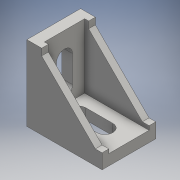
# Autodesk Inventor part: KeGoc2020_SuaLai
Saved by Autodesk Inventor 2016 (Build 200138000, 138)
## iProperties
Created: 2020-11-23
Part Number: KeGoc2020_SuaLai
Material: Generic
Document SubType Name: Modeling
Designer: TG
Density: 1 g/cm^3
Appearance: Default
Author: TG
Autodesk Inventor part; units mm, degrees
ref_plane "YZ Plane" through (0, 0, 0) normal (1, 0, 0) x (0, 1, 0)
ref_plane "XZ Plane" through (0, 0, 0) normal (0, 1, 0) x (-1, 0, 0)
ref_plane "XY Plane" through (0, 0, 0) normal (0, 0, 1) x (1, 0, 0)
sketch "Sketch1" plane through (0, 0, 0) normal (0, 0, 1) x (1, 0, 0)
  line L0 (-17.8, 7.2667) -> (10.2, 7.2667)
  line L1 (10.2, 7.2667) -> (10.2, -12.7333)
  line L2 (10.2, -12.7333) -> (-17.8, -12.7333)
  line L3 (-17.8, -12.7333) -> (-17.8, 7.2667)
  point P0 (0, 0)
  dimension "d0" = 20
  dimension "d1" = 28
  constraints: 8 end point, 2 parallel, 1 horizontal, 1 perpendicular
  measures "d0" distance of L0.end L1.end
  measures "d1" distance of L1.end L2.end
extrude "Extrusion1" add sketch "Sketch1" along normal blind 4
sketch "Sketch2" plane through (0, 0, 4) normal (0, 0, 1) x (1, 0, 0)
  line L0 (10.2, 7.2667) -> (-17.8, 7.2667) projected
  line L1 (-17.8, 7.2667) -> (-17.8, -12.7333) projected
  line L2 (-17.8, -12.7333) -> (10.2, -12.7333) projected
  line L3 (10.2, -12.7333) -> (10.2, 7.2667) projected
  line L4 (-17.8, 7.2667) -> (-17.8, -12.7333) projected
  line L5 (-17.8, -2.7333) -> (10.2, -2.7333) construction
  line L6 (10.2, -12.7333) -> (10.2, 7.2667) projected
  line L7 (-8.8, -2.7333) -> (1.2, -2.7333) construction
  line L8 (-8.8, -5.7333) -> (1.2, -5.7333)
  line L9 (1.2, 0.2667) -> (-8.8, 0.2667)
  arc A0 (-8.8, 0.2667) -> (-8.8, -5.7333) centre (-8.8, -2.7333) ccw
  arc A1 (1.2, -5.7333) -> (1.2, 0.2667) centre (1.2, -2.7333) ccw
  point P0 (0, 0)
  point P1 (-3.8, -2.7333)
  dimension "d4" = 10
  dimension "d5" = 6
  dimension "d6" = 9
  constraints: 10 end point, 4 point on circle, 4 tangent, 3 midpoint, 2 centre point, 2 point on line, 1 parallel
  measures "d4" distance of L7.start L7.end
  measures "d5" diameter of A1
  measures "d6" distance of L5.end L7.end
extrude "Extrusion2" cut sketch "Sketch2" against normal blind 30 contours A0 L9 A1 L8
sketch "Sketch3" plane through (0, 0, 4) normal (0, 0, 1) x (1, 0, 0)
  arc A0 (1.2, -5.7333) -> (1.2, 0.2667) centre (1.2, -2.7333) ccw projected
  line L0 (1.2, -5.7333) -> (-8.8, -5.7333) projected
  arc A1 (-8.8, 0.2667) -> (-8.8, -5.7333) centre (-8.8, -2.7333) ccw projected
  line L1 (-8.8, 0.2667) -> (1.2, 0.2667) projected
  line L2 (10.2, 7.2667) -> (-17.8, 7.2667) projected
  line L3 (-17.8, 7.2667) -> (-17.8, -12.7333) projected
  line L4 (-17.8, -12.7333) -> (10.2, -12.7333) projected
  line L5 (10.2, -12.7333) -> (10.2, 7.2667) projected
  line L6 (-17.8, -12.7333) -> (-17.8, 7.2667) projected
  line L7 (-17.8, 7.2667) -> (-13.8, 7.2667)
  line L8 (-13.8, 7.2667) -> (-13.8, -12.7333)
  line L9 (-13.8, -12.7333) -> (-17.8, -12.7333)
  line L10 (-17.8, -12.7333) -> (-17.8, 7.2667)
  point P0 (0, 0)
  dimension "d9" = 4
  constraints: 8 end point, 2 parallel, 1 horizontal, 1 perpendicular, 1 point on line
  measures "d9" distance between parallel lines of L8 L3
extrude "Extrusion3" add sketch "Sketch3" along normal blind 24 contours L8 L4 L3 L2
sketch "Sketch4" plane through (-17.8, -12.7333, 0) normal (-1, 0, 0) x (0, 0, 1)
  line L0 (0, 0) -> (0, 20) projected
  line L1 (0, 0) -> (28, 0) projected
  line L2 (28, 20) -> (28, 0) projected
  line L3 (0, 20) -> (28, 20) projected
  line L4 (0, 0) -> (0, 20) projected
  line L5 (0, 10) -> (28, 10) construction
  line L6 (28, 0) -> (28, 20) projected
  line L7 (9, 10) -> (19, 10) construction
  line L8 (9, 7) -> (19, 7)
  line L9 (19, 13) -> (9, 13)
  arc A0 (9, 13) -> (9, 7) centre (9, 10) ccw
  arc A1 (19, 7) -> (19, 13) centre (19, 10) ccw
  point P0 (0, 12.7333)
  point P1 (14, 10)
  dimension "d12" = 10
  dimension "d13" = 6
  dimension "d14" = 9
  constraints: 10 end point, 4 point on circle, 4 tangent, 3 midpoint, 2 centre point, 2 point on line, 1 parallel
  measures "d12" distance of L7.start L7.end
  measures "d13" diameter of A1
  measures "d14" distance of L5.end L7.end
extrude "Extrusion4" cut sketch "Sketch4" against normal blind 24 contours A0 L9 A1 L8
sketch "Sketch5" plane through (-17.8, -12.7333, 0) normal (-1, 0, 0) x (0, 0, 1)
  arc A0 (19, 7) -> (19, 13) centre (19, 10) ccw projected
  line L0 (19, 7) -> (9, 7) projected
  arc A1 (9, 13) -> (9, 7) centre (9, 10) ccw projected
  line L1 (9, 13) -> (19, 13) projected
  line L2 (0, 0) -> (0, 20) projected
  line L3 (0, 0) -> (28, 0) projected
  line L4 (28, 20) -> (28, 0) projected
  line L5 (0, 20) -> (28, 20) projected
  line L6 (27, 12.9) -> (26, 12.9)
  line L7 (26, 12.9) -> (26, 7.1)
  line L8 (26, 7.1) -> (27, 7.1)
  line L9 (27, 7.1) -> (27, 12.9)
  line L10 (28, 0) -> (28, 20) projected
  line L11 (28, 10) -> (34.771, 10) construction
  point P0 (0, 12.7333)
  dimension "d17" = 1
  dimension "d18" = 5.8
  dimension "d19" = 1
  constraints: 10 end point, 2 horizontal, 2 parallel, 1 midpoint, 1 perpendicular, 1 other
  measures "d17" distance between parallel lines of L7 L9
  measures "d18" distance between parallel lines of L8 L6
  measures "d19" distance between parallel lines of L4 L9
extrude "Extrusion5" add sketch "Sketch5" along normal blind 1 contours L9 L8 L7 L6
sketch "Sketch6" plane through (0, 0, 0) normal (0, 0, -1) x (-1, 0, 0)
  arc A0 (-1.2, 0.2667) -> (-1.2, -5.7333) centre (-1.2, -2.7333) ccw projected
  line L0 (-1.2, 0.2667) -> (8.8, 0.2667) projected
  arc A1 (8.8, -5.7333) -> (8.8, 0.2667) centre (8.8, -2.7333) ccw projected
  line L1 (8.8, -5.7333) -> (-1.2, -5.7333) projected
  line L2 (17.8, 7.2667) -> (-10.2, 7.2667) projected
  line L3 (-10.2, 7.2667) -> (-10.2, -12.7333) projected
  line L4 (-10.2, -12.7333) -> (17.8, -12.7333) projected
  line L5 (17.8, -12.7333) -> (17.8, 7.2667) projected
  line L6 (-9.2, -5.6333) -> (-8.2, -5.6333)
  line L7 (-8.2, -5.6333) -> (-8.2, 0.1667)
  line L8 (-8.2, 0.1667) -> (-9.2, 0.1667)
  line L9 (-9.2, 0.1667) -> (-9.2, -5.6333)
  line L10 (-10.2, -2.7333) -> (-3.3022, -2.7333) construction
  point P0 (0, 0)
  dimension "d22" = 1
  dimension "d23" = 5.8
  dimension "d24" = 1
  constraints: 10 end point, 2 horizontal, 2 parallel, 1 midpoint, 1 perpendicular, 1 other
  measures "d22" distance between parallel lines of L7 L9
  measures "d23" distance between parallel lines of L8 L6
  measures "d24" distance between parallel lines of L3 L9
extrude "Extrusion6" add sketch "Sketch6" along normal blind 1 contours L9 L8 L7 L6
sketch "Sketch7" plane through (-17.8, -12.7333, 0) normal (0, -1, 0) x (1, 0, 0)
  line L0 (28, 0) -> (0, 0) projected
  line L1 (28, 0) -> (28, 4) projected
  line L2 (4, 4) -> (28, 4) projected
  line L3 (4, 4) -> (4, 28) projected
  line L4 (0, 28) -> (4, 28) projected
  line L5 (0, 0) -> (0, 28) projected
  line L6 (4, 28) -> (5.5, 28)
  line L7 (5.5, 28) -> (5.5, 25.5)
  line L8 (28, 4) -> (28, 5.5)
  line L9 (28, 5.5) -> (25.5, 5.5)
  line L10 (25.5, 5.5) -> (5.5, 25.5)
  point P0 (17.8, 0)
  dimension "d27" = 1.5
  dimension "d28" = 2.5
  dimension "d29" = 1.5
  dimension "d30" = 2.5
  constraints: 10 end point, 2 perpendicular, 1 horizontal, 1 vertical
  measures "d27" distance of L3.end L6.end
  measures "d28" distance of L6.end L7.end
  measures "d29" distance of L1.end L8.end
  measures "d30" distance of L8.end L9.end
extrude "Extrusion7" add sketch "Sketch7" against normal blind 2.5 contours L2 L3 L6 L7 L10 L9 L8
sketch "Sketch8" plane through (-17.8, 7.2667, 0) normal (0, 1, 0) x (1, 0, 0)
  line L0 (0, 0) -> (28, 0) projected
  line L1 (0, 0) -> (0, -28) projected
  line L2 (4, -28) -> (0, -28) projected
  line L3 (4, -4) -> (4, -28) projected
  line L4 (28, -4) -> (4, -4) projected
  line L5 (28, 0) -> (28, -4) projected
  line L6 (4, -4) -> (4, -28) projected
  line L7 (28, -5.5) -> (28, -4) projected
  line L8 (4, -4) -> (28, -4) projected
  line L9 (4, -28) -> (4, -4) projected
  line L10 (4, -28) -> (5.5, -28) projected
  line L11 (5.5, -28) -> (5.5, -25.5) projected
  line L12 (5.5, -25.5) -> (25.5, -5.5) projected
  line L13 (25.5, -5.5) -> (28, -5.5) projected
  point P0 (17.8, 0)
extrude "Extrusion8" add sketch "Sketch8" against normal blind 2.5 contours L7 L13 L12 L11 L10 L3 L4
body "Solid1"
